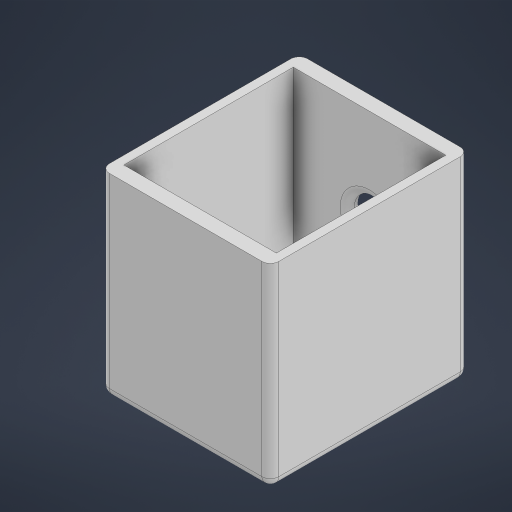
# Autodesk Inventor part: shooter-comp
Saved by Autodesk Inventor 2023 (Build 270158030, 158C)
## iProperties
Created: 2022-05-15
Part Number: shooter-comp
Material: Generic
Document SubType Name: Modeling
Designer: jayso
Density: 1 g/cm^3
Appearance: Default
Author: jayso
Autodesk Inventor part; units mm, degrees
ref_plane "YZ Plane" through (0, 0, 0) normal (1, 0, 0) x (0, 1, 0)
ref_plane "XZ Plane" through (0, 0, 0) normal (0, 1, 0) x (-1, 0, 0)
ref_plane "XY Plane" through (0, 0, 0) normal (0, 0, 1) x (1, 0, 0)
sketch "Sketch2" plane through (0, 0, 0) normal (0, 1, 0) x (-1, 0, 0)
  line L0 (57.5, 58.5) -> (-42.5, 58.5)
  line L1 (-42.5, 58.5) -> (-42.5, -58.5)
  line L2 (-42.5, -58.5) -> (57.5, -58.5)
  line L3 (57.5, -58.5) -> (57.5, 58.5)
  point P0 (0, 0)
  dimension "d0" = 117
  dimension "d1" = 100
  dimension "d2" = 58.5
  dimension "d3" = 57.5
  constraints: 8 end point, 2 parallel, 1 horizontal, 1 perpendicular
  measures "d0" distance between parallel lines of L2 L0
  measures "d1" distance of L1.end L2.end
  measures "d2" vertical distance of point (0, 0) L2.end
  measures "d3" horizontal distance of point (0, 0) L0.start
extrude "Extrusion1" add sketch "Sketch2" along normal blind 115
sketch "Sketch3" plane through (-57.5, 0, -58.5) normal (-1, 0, 0) x (0, 0, 1)
  circle A0 centre (58.5, 57.5) radius 4
  line L0 (0, 115) -> (117, 115) projected
  line L1 (0, 0) -> (0, 115) projected
  point P0 (58.5, 0)
  point P1 (58.5, 115)
  dimension "d6" = 8
  dimension "d7" = 57.5
  dimension "d8" = 58.5
  constraints: 1 centre point, 1 midpoint
  measures "d6" diameter of A0
  measures "d7" distance of point (58.5, 115) A0.centre
  measures "d8" distance from line of L1 A0.centre
extrude "Extrusion2" add sketch "Sketch3" along normal blind 34
sketch "Sketch4" plane through (0, 115, 0) normal (0, 1, 0) x (1, 0, 0)
  line L0 (-52.5, 50) -> (37.5, 50)
  line L1 (37.5, 50) -> (37.5, -50)
  line L2 (37.5, -50) -> (-52.5, -50)
  line L3 (-52.5, -50) -> (-52.5, 50)
  line L4 (-57.5, 58.5) -> (-57.5, -58.5) projected
  line L5 (-57.5, -58.5) -> (42.5, -58.5) projected
  point P0 (0, 0)
  dimension "d11" = 90
  dimension "d12" = 5
  dimension "d13" = 100
  dimension "d14" = 8.5
  constraints: 8 end point, 2 parallel, 1 horizontal, 1 perpendicular
  measures "d11" distance of L0.start L0.end
  measures "d12" distance between parallel lines of L4 L3
  measures "d13" distance of L0.end L1.end
  measures "d14" distance from line of L5 L1.end
extrude "Extrusion3" cut sketch "Sketch4" against normal blind 110
sketch "Sketch5" plane through (42.5, 0, -58.5) normal (0, 0, -1) x (-1, 0, 0)
  circle A0 centre (50, 57.5) radius 12.5
  line L0 (0, 115) -> (100, 115) projected
  line L1 (100, 0) -> (100, 115) projected
  point P0 (42.5, 0)
  point P1 (50, 115)
  dimension "d17" = 25
  dimension "d18" = 57.5
  dimension "d19" = 50
  constraints: 1 centre point, 1 midpoint
  measures "d17" diameter of A0
  measures "d18" distance of point (50, 115) A0.centre
  measures "d19" distance from line of L1 A0.centre
extrude "Extrusion4" cut sketch "Sketch5" against normal blind 10
fillet "Fillet1" radius 5 10 edges at (-7.5, 0, -58.5) (-57.5, 57.5, -58.5) (-57.5, 0, 0) (-7.5, 0, 58.5) (-57.5, 57.5, 58.5) (42.5, 57.5, 58.5) (42.5, 0, 0) (42.5, 57.5, -58.5) (5, 57.5, -58.5) (5, 57.5, -50)
body "Solid1"
